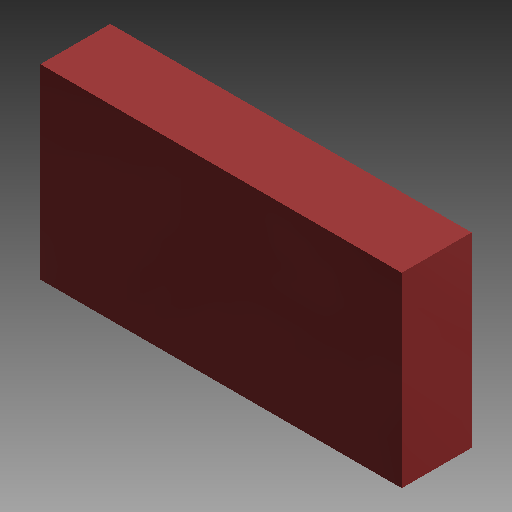
# Autodesk Inventor part: 0.1r
Saved by Autodesk Inventor 2018.2 (Build 222227000, 227)
## iProperties
Part Number: 0.1r
Material: Generic
Document SubType Name: Modeling
Designer: autocad
Appearance: R1206, 0.1r
Author: autocad
Autodesk Inventor part; units mm, degrees
ref_plane "YZ Plane" through (0, 0, 0) normal (1, 0, 0) x (0, 1, 0)
ref_plane "XZ Plane" through (0, 0, 0) normal (0, 1, 0) x (-1, 0, 0)
ref_plane "XY Plane" through (0, 0, 0) normal (0, 0, 1) x (1, 0, 0)
sketch "R1206, 0.1r_248" plane through (0, 0, 0) normal (0, 0, 1) x (1, 0, 0)
  line L0 (1.55, 0.8) -> (1.55, -0.8)
  line L1 (1.55, -0.8) -> (-1.55, -0.8)
  line L2 (-1.55, -0.8) -> (-1.55, 0.8)
  line L3 (-1.55, 0.8) -> (1.55, 0.8)
  constraints: 8 end point
extrude "Extrusion1" add sketch "R1206, 0.1r_248" along normal blind 0.6
body "Solid1"
